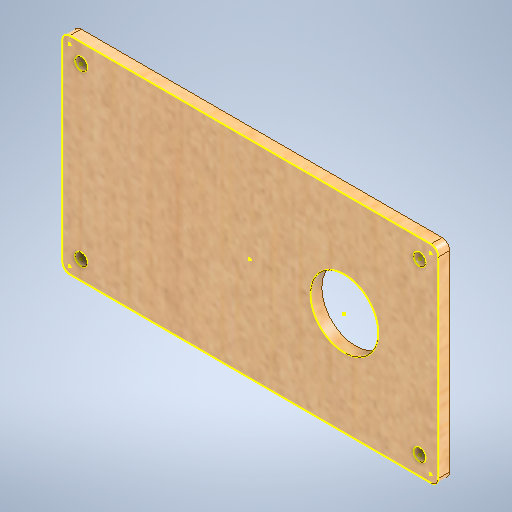
# Autodesk Inventor part: xx_plate_nomotor
Saved by Autodesk Inventor 2025.1 (Build 291241000, 241)
## iProperties
Created: 2024-12-04
Part Number: xx_plate_nomotor
Material: 一般
Document SubType Name: Modeling
Designer: yuki0520
Density: 1 g/cm^3
Appearance: イエロー パイン材 - 硬質 塗装 抑えた光沢
Author: yuki0520
Autodesk Inventor part; units mm, degrees
ref_plane "YZ Plane" through (0, 0, 0) normal (1, 0, 0) x (0, 1, 0)
ref_plane "XZ Plane" through (0, 0, 0) normal (0, 1, 0) x (-1, 0, 0)
ref_plane "XY Plane" through (0, 0, 0) normal (0, 0, 1) x (1, 0, 0)
sketch "スケッチ1" plane through (0, 0, 0) normal (0, 0, 1) x (1, 0, 0)
  line L0 (50, -27.5) -> (-50, -27.5)
  line L1 (-50, -27.5) -> (-50, 27.5)
  line L2 (-50, 27.5) -> (50, 27.5)
  line L3 (50, 27.5) -> (50, -27.5)
  line L4 (50, -27.5) -> (-50, 27.5) construction
  line L5 (-50, -27.5) -> (50, 27.5) construction
  circle A0 centre (0, 0) radius 25
  line L6 (-50, 0) -> (50, 0)
  circle A1 centre (25, 0) radius 9
  circle A2 centre (-25, 0) radius 12.5
  circle A3 centre (-25, 0) radius 17.5
  circle A4 centre (-25, 17.5) radius 2.05
  circle A5 centre (-42.5, 0) radius 2.05
  circle A6 centre (-25, -17.5) radius 2.05
  circle A7 centre (-7.5, 0) radius 2.05
  dimension "d5" = 35
  dimension "d0" = 100
  dimension "d1" = 55
  dimension "d2" = 50
  dimension "d3" = 18
  dimension "d4" = 25
  dimension "d6" = 4.1
  dimension "d9" = 360
  dimension "d11" = 25
  constraints: 14 end point, 7 centre point, 4 midpoint, 2 coincident, 2 parallel, 2 point on circle, 2 point on line, 1 horizontal, 1 perpendicular, 1 vertical alignment, 11 other
  measures "d0" distance of L1.end L2.end
  measures "d1" distance of L0.end L1.end
  measures "d2" diameter of A0
  measures "d3" diameter of A1
  measures "d4" diameter of A2
  measures "d6" diameter of A4
  measures "d11" distance from line of L1 A4.centre
extrude "押し出し1" add sketch "スケッチ1" along normal blind 3 contours L0 L1 L6 A5 A3 A6 A0 A1 L3 | L6 A1 A0 A3 A4 A5 L1 L2 L3 | A5 A3 L6 | L6 A3 A5 | A1 L6 A7 A3 A0 | A0 A3 A7 L6 A1 | A3 A5 L6 | L6 A5 A3 | A3 A4 A0 A2 L6 A5 | A5 L6 A2 A0 A3 A6 | A3 A7 L6 A2 A0 | A0 A2 L6 A7 A3 | A4 A3 | A3 A4 | A6 A3 | A3 A6 | A7 A3 L6 | L6 A3 A7 | A2 L6 A0 | A0 L6 A2 | A3 L6 A7 | A2 L6 A0 | A0 L6 A2 | A7 L6 A3
sketch "スケッチ2" plane through (0, 0, 3) normal (0, 0, 1) x (1, 0, 0)
  line L0 (50, 27.5) -> (-50, 27.5) projected
  line L1 (-50, 27.5) -> (-50, -27.5) projected
  line L2 (-50, -27.5) -> (50, -27.5) projected
  line L3 (50, -27.5) -> (50, 27.5) projected
  circle A0 centre (25, 0) radius 9 projected
  line L4 (-45, 22.5) -> (45, 22.5)
  line L5 (45, 22.5) -> (45, -22.5)
  line L6 (45, -22.5) -> (-45, -22.5)
  line L7 (-45, -22.5) -> (-45, 22.5)
  point P0 (0, 0)
  dimension "d14" = 5
  constraints: 8 end point, 4 coincident, 3 other
  measures "d14" distance between parallel lines of L0 L4
hole "穴1" at (-45, 22.5, 3) at (-45, -22.5, 3) at (45, -22.5, 3) at (45, 22.5, 3) direction (0, 0, -1) diameter 3.2 end through all
fillet "フィレット1" radius 2 4 edges at (-50, 27.5, 1.5) (50, 27.5, 1.5) (50, -27.5, 1.5) (-50, -27.5, 1.5)
sketch "スケッチ3" plane through (0, 0, 3) normal (0, 0, 1) x (1, 0, 0)
  arc A0 (-50, -25.5) -> (-48, -27.5) centre (-48, -25.5) ccw projected
  line L0 (-48, -27.5) -> (48, -27.5) projected
  arc A1 (48, -27.5) -> (50, -25.5) centre (48, -25.5) ccw projected
  line L1 (50, -25.5) -> (50, 25.5) projected
  arc A2 (50, 25.5) -> (48, 27.5) centre (48, 25.5) ccw projected
  line L2 (48, 27.5) -> (-48, 27.5) projected
  arc A3 (-48, 27.5) -> (-50, 25.5) centre (-48, 25.5) ccw projected
  line L3 (-50, 25.5) -> (-50, -25.5) projected
  circle A4 centre (45, 22.5) radius 1.6 projected
  circle A5 centre (45, -22.5) radius 1.6 projected
  circle A6 centre (-45, -22.5) radius 1.6 projected
  circle A7 centre (-45, 22.5) radius 1.6 projected
  circle A8 centre (25, 0) radius 9 projected
  point P0 (0, 0)
equation "\"d11\" = -0.5 * d2 + 0.5 * d0"
